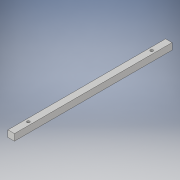
# Autodesk Inventor part: height 460
Saved by Autodesk Inventor 2019 (Build 230136000, 136)
## iProperties
Created: 2021-03-22
Part Number: height 460
Material: Generic
Document SubType Name: Modeling
Designer: User
Density: 1 g/cm^3
Appearance: Default
Author: User
Autodesk Inventor part; units mm, degrees
ref_plane "YZ Plane" through (0, 0, 0) normal (1, 0, 0) x (0, 1, 0)
ref_plane "XZ Plane" through (0, 0, 0) normal (0, 1, 0) x (-1, 0, 0)
ref_plane "XY Plane" through (0, 0, 0) normal (0, 0, 1) x (1, 0, 0)
sketch "Sketch1" plane through (0, 0, 0) normal (0, 1, 0) x (-1, 0, 0)
  line L0 (19, 213.7275) -> (0, 213.7275)
  line L1 (0, 213.7275) -> (0, -246.2725)
  line L2 (0, -246.2725) -> (19, -246.2725)
  line L3 (19, -246.2725) -> (19, 213.7275)
  point P0 (0, 0)
  dimension "d0" = 19
  dimension "d1" = 460
  dimension "d2" = 19
  dimension "d3" = 213.7275
  constraints: 8 end point, 2 parallel, 1 horizontal, 1 perpendicular
  measures "d0" distance between parallel lines of L3 L1
  measures "d1" distance between parallel lines of L2 L0
  measures "d2" distance from line of point (0, 0) L3
  measures "d3" distance from line of point (0, 0) L0
extrude "Extrusion1" add sketch "Sketch1" along normal mid plane 19
sketch "Sketch2" plane through (0, 9.5, 0) normal (0, 1, 0) x (1, 0, 0)
  circle A0 centre (-9.5, -163.7275) radius 4
  circle A1 centre (-9.5, 196.2725) radius 4
  line L0 (-19, -213.7275) -> (0, -213.7275) projected
  line L1 (0, 246.2725) -> (-19, 246.2725) projected
  line L2 (-19, 246.2725) -> (-19, -213.7275) projected
  line L3 (0, -213.7275) -> (0, 246.2725) projected
  point P0 (0, 0)
  dimension "d6" = 50
  dimension "d7" = 50
  dimension "d8" = 9.5
  dimension "d9" = 9.5
  dimension "d10" = 8
  dimension "d11" = 8
  constraints: 2 centre point
  measures "d6" distance from line of A0.centre L0
  measures "d7" distance from line of L1 A1.centre
  measures "d8" distance from line of L2 A0.centre
  measures "d9" distance from line of L3 A1.centre
  measures "d10" diameter of A0
  measures "d11" diameter of A1
extrude "Extrusion2" cut sketch "Sketch2" against normal blind 19 contours A0 | A1
body "Solid1"
